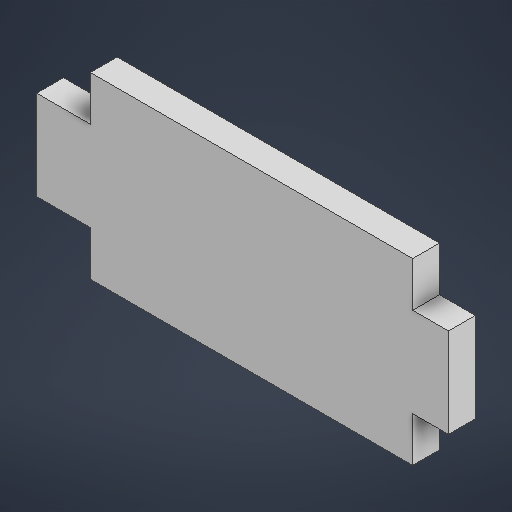
# Autodesk Inventor part: Battary_holder_part3
Saved by Autodesk Inventor 2027 (Build 310192000, 192)
## iProperties
Created: 2026-06-03
Part Number: Battary_holder_part3
Material: Generic
Document SubType Name: Modeling
Designer: alexy
Density: 1 g/cm^3
Appearance: Default
Author: alexy
Autodesk Inventor part; units mm, degrees
ref_plane "YZ Plane" through (0, 0, 0) normal (1, 0, 0) x (0, 1, 0)
ref_plane "XZ Plane" through (0, 0, 0) normal (0, 1, 0) x (-1, 0, 0)
ref_plane "XY Plane" through (0, 0, 0) normal (0, 0, 1) x (1, 0, 0)
sketch "Sketch1" plane through (0, 0, 0) normal (0, 0, 1) x (1, 0, 0)
  line L0 (0, 0) -> (36, 0)
  line L1 (36, 0) -> (36, 20)
  line L2 (36, 20) -> (0, 20)
  line L3 (0, 20) -> (0, 0)
  line L4 (-6, 15) -> (0, 15)
  line L5 (0, 15) -> (0, 5)
  line L6 (0, 5) -> (-6, 5)
  line L7 (-6, 5) -> (-6, 15)
  line L8 (-6, 15) -> (0, 5) construction
  line L9 (0, 15) -> (-6, 5) construction
  line L10 (40, 15) -> (36, 15)
  line L11 (36, 15) -> (36, 5)
  line L12 (36, 5) -> (40, 5)
  line L13 (40, 5) -> (40, 15)
  line L14 (40, 15) -> (36, 5) construction
  line L15 (36, 15) -> (40, 5) construction
  point P0 (-3, 10)
  point P1 (38, 10)
  dimension "d0" = 36
  dimension "d1" = 20
  dimension "d2" = 4
  dimension "d3" = 6
  dimension "d4" = 10
  dimension "d5" = 10
  constraints: 32 end point, 6 parallel, 4 midpoint, 3 horizontal, 3 perpendicular, 2 horizontal alignment, 2 point on line
  measures "d0" distance of L1.end L2.end
  measures "d1" distance of L0.end L1.end
  measures "d2" distance of L11.end L12.end
  measures "d3" distance of L5.end L6.end
  measures "d4" distance of L12.end L10.start
  measures "d5" vertical distance of L0.end point (38, 10)
extrude "Extrusion1" add sketch "Sketch1" along normal blind 3
body "Solid1"
